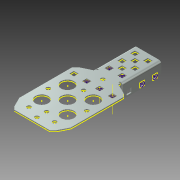
# Autodesk Inventor part: VEX_Bracket
Saved by Autodesk Inventor 2013 (Build 170138000, 138)
## iProperties
Created: 2011-03-28
Part Number: VEX_Bracket
Material: Aluminum-6061
Document SubType Name: Sheet Metal
Designer: Phillip
Density: 2.71 g/cm^3
Sheet Metal Rule: Default
Mass: 13.8705 g
Surface Area: 99.2536 cm^2
Volume: 5.11826 cm^3
Flat Pattern Width: 5.08 cm
Flat Pattern Length: 11.43 cm
Flat Pattern Area: 58.0644 cm^2
Sheet Metal Width: 2.000 in
Sheet Metal Length: 4.500 in
Sheet Metal Area: 9.000 in^2
Author: Phillip
Autodesk Inventor part; units mm, degrees
ref_plane "YZ Plane" through (0, 0, 0) normal (1, 0, 0) x (0, 1, 0)
ref_plane "XZ Plane" through (0, 0, 0) normal (0, 1, 0) x (-1, 0, 0)
ref_plane "XY Plane" through (0, 0, 0) normal (0, 0, 1) x (1, 0, 0)
sketch "Sketch1" plane through (0, 0, 0) normal (0, 0, 1) x (1, 0, 0)
  line L0 (-3.175, 3.175) -> (-7.9375, 12.7)
  line L1 (-3.175, 3.175) -> (0, 0)
  line L2 (0, 0) -> (34.925, 0)
  line L3 (38.1, 3.175) -> (34.925, 0)
  line L4 (38.1, 3.175) -> (42.8625, 12.7)
  line L5 (42.8625, 12.7) -> (42.8625, 65.0133)
  line L6 (39.6875, 68.1883) -> (42.8625, 65.0133)
  line L7 (39.6875, 68.1883) -> (29.5402, 73.025)
  line L8 (29.5402, 73.025) -> (29.5402, 114.3)
  line L9 (29.5402, 114.3) -> (5.3848, 114.3)
  line L10 (5.3848, 114.3) -> (5.3848, 73.025)
  line L11 (-4.7625, 68.1883) -> (5.3848, 73.025)
  line L12 (-4.7625, 68.1883) -> (-7.9375, 65.0133)
  line L13 (-7.9375, 12.7) -> (-7.9375, 65.0133)
  line L14 (19.7739, 99.2886) -> (19.7739, 103.9114)
  line L15 (15.1511, 99.2886) -> (19.7739, 99.2886)
  line L16 (15.1511, 103.9114) -> (15.1511, 99.2886)
  line L17 (19.7739, 103.9114) -> (15.1511, 103.9114)
  line L18 (13.4239, 105.6386) -> (13.4239, 110.2614)
  line L19 (8.8011, 105.6386) -> (13.4239, 105.6386)
  line L20 (8.8011, 110.2614) -> (8.8011, 105.6386)
  line L21 (13.4239, 110.2614) -> (8.8011, 110.2614)
  line L22 (26.1239, 105.6386) -> (26.1239, 110.2614)
  line L23 (21.5011, 105.6386) -> (26.1239, 105.6386)
  line L24 (21.5011, 110.2614) -> (21.5011, 105.6386)
  line L25 (26.1239, 110.2614) -> (21.5011, 110.2614)
  line L26 (26.1239, 58.0136) -> (26.1239, 62.6364)
  line L27 (21.5011, 58.0136) -> (26.1239, 58.0136)
  line L28 (21.5011, 62.6364) -> (21.5011, 58.0136)
  line L29 (26.1239, 62.6364) -> (21.5011, 62.6364)
  line L30 (38.8239, 58.0136) -> (38.8239, 62.6364)
  line L31 (34.2011, 58.0136) -> (38.8239, 58.0136)
  line L32 (34.2011, 62.6364) -> (34.2011, 58.0136)
  line L33 (38.8239, 62.6364) -> (34.2011, 62.6364)
  circle A0 centre (30.1625, 47.625) radius 6.35
  circle A1 centre (4.7625, 47.625) radius 6.35
  circle A2 centre (4.7625, 22.225) radius 6.35
  circle A3 centre (30.1625, 22.225) radius 6.35
  circle A4 centre (17.4625, 34.925) radius 6.35
  circle A5 centre (17.4625, 69.85) radius 2.0701
  circle A6 centre (17.4625, 50.8) radius 2.0701
  circle A7 centre (17.4625, 14.2875) radius 2.0701
  circle A8 centre (17.4625, 4.7625) radius 2.0701
  circle A9 centre (4.7625, 9.525) radius 2.0701
  circle A10 centre (30.1625, 9.525) radius 2.0701
  circle A11 centre (-1.5875, 34.925) radius 2.0701
  circle A12 centre (36.5125, 34.925) radius 2.0701
  line L34 (13.4239, 58.0136) -> (13.4239, 62.6364)
  line L35 (8.8011, 58.0136) -> (13.4239, 58.0136)
  line L36 (8.8011, 62.6364) -> (8.8011, 58.0136)
  line L37 (13.4239, 62.6364) -> (8.8011, 62.6364)
  line L38 (0.7239, 58.0136) -> (0.7239, 62.6364)
  line L39 (-3.8989, 58.0136) -> (0.7239, 58.0136)
  line L40 (-3.8989, 62.6364) -> (-3.8989, 58.0136)
  line L41 (0.7239, 62.6364) -> (-3.8989, 62.6364)
  line L42 (26.1239, 92.9386) -> (26.1239, 97.5614)
  line L43 (21.5011, 92.9386) -> (26.1239, 92.9386)
  line L44 (21.5011, 97.5614) -> (21.5011, 92.9386)
  line L45 (26.1239, 97.5614) -> (21.5011, 97.5614)
  line L46 (13.4239, 92.9386) -> (13.4239, 97.5614)
  line L47 (8.8011, 92.9386) -> (13.4239, 92.9386)
  line L48 (8.8011, 97.5614) -> (8.8011, 92.9386)
  line L49 (13.4239, 97.5614) -> (8.8011, 97.5614)
  line L50 (26.1239, 80.2386) -> (26.1239, 84.8614)
  line L51 (21.5011, 80.2386) -> (26.1239, 80.2386)
  line L52 (21.5011, 84.8614) -> (21.5011, 80.2386)
  line L53 (26.1239, 84.8614) -> (21.5011, 84.8614)
  line L54 (13.4239, 80.2386) -> (13.4239, 84.8614)
  line L55 (8.8011, 80.2386) -> (13.4239, 80.2386)
  line L56 (8.8011, 84.8614) -> (8.8011, 80.2386)
  line L57 (13.4239, 84.8614) -> (8.8011, 84.8614)
  line L58 (19.7739, 86.5886) -> (19.7739, 91.2114)
  line L59 (15.1511, 86.5886) -> (19.7739, 86.5886)
  line L60 (15.1511, 91.2114) -> (15.1511, 86.5886)
  line L61 (19.7739, 91.2114) -> (15.1511, 91.2114)
  circle A13 centre (11.1125, 107.95) radius 2.3114
  circle A14 centre (11.1125, 95.25) radius 2.3114
  circle A15 centre (11.1125, 82.55) radius 2.3114
  circle A16 centre (23.8125, 107.95) radius 2.3114
  circle A17 centre (23.8125, 95.25) radius 2.3114
  circle A18 centre (23.8125, 82.55) radius 2.3114
  circle A19 centre (-1.5875, 60.325) radius 2.3114
  circle A20 centre (11.1125, 60.325) radius 2.3114
  circle A21 centre (23.8125, 60.325) radius 2.3114
  circle A22 centre (36.5125, 60.325) radius 2.3114
  dimension "d8" = 12.7
  dimension "d9" = 12.7
  dimension "d10" = 12.7
  dimension "d12" = 6.35
  dimension "d13" = 24.1554
  dimension "d14" = 41.275
  dimension "d15" = 114.3
  dimension "d16" = 50.8
  dimension "d17" = 4.1402
  dimension "d18" = 4.6228
  dimension "d19" = 4.6228
  measures "d8" distance of A13.centre A14.centre
  measures "d9" distance of A13.centre A16.centre
  measures "d10" distance of A19.centre A20.centre
  measures "d12" distance from line of A13.centre L9
  measures "d13" distance of L8.end L10.start
  measures "d14" distance of L8.start L8.end
  measures "d15" vertical distance of L3.end L8.end
  measures "d16" distance between parallel lines of L5 L13
  measures "d17" diameter of A11
  measures "d18" distance of L57.end L56.end
  measures "d19" distance of L57.start L57.end
extrude "Plate1" add sketch "Sketch1" along normal blind 1.1684
sketch "Sketch2" plane through (29.5402, 73.025, 0) normal (1, 0, 0) x (0, 0, -1)
  line L0 (0, 41.275) -> (12.7, 41.275)
  line L1 (12.7, 41.275) -> (12.7, 3.175)
  line L2 (12.7, 3.175) -> (0, 3.175)
  line L3 (0, 3.175) -> (0, 41.275)
  point P0 (0, -73.025)
  dimension "d21" = 12.7
  dimension "d22" = 38.1
  measures "d21" distance of L1.end L2.end
  measures "d22" distance of L0.end L1.end
sheet face with bend "Face2" sketch "Sketch2" thickness 1.1684 toward (1, 0, 0) bend radius 1.1684 relief straight relief width 1.1684 relief depth 0.5842
bend "Bend1"
sketch "Sketch3" plane through (5.3848, 73.025, 0) normal (-1, 0, 0) x (0, 0, 1)
  line L0 (0, 41.275) -> (-12.7, 41.275)
  line L1 (-12.7, 41.275) -> (-12.7, 3.175)
  line L2 (-12.7, 3.175) -> (0, 3.175)
  line L3 (0, 3.175) -> (0, 41.275)
  point P0 (0, -73.025)
  dimension "d28" = 12.7
  dimension "d29" = 38.1
  measures "d28" distance of L2.end L1.end
  measures "d29" distance of L1.end L0.end
sheet face with bend "Face3" sketch "Sketch3" thickness 1.1684 toward (-1, 0, 0) bend radius 1.1684 relief straight relief width 1.1684 relief depth 0.5842
bend "Bend2"
sketch "Sketch4" plane through (30.7086, 73.025, 0) normal (1, 0, 0) x (0, 0, -1)
  line L0 (1.1684, 41.275) -> (1.1684, 3.175)
  line L1 (11.2522, 37.2364) -> (6.6294, 37.2364)
  line L2 (11.2522, 32.6136) -> (11.2522, 37.2364)
  line L3 (6.6294, 32.6136) -> (11.2522, 32.6136)
  line L4 (6.6294, 37.2364) -> (6.6294, 32.6136)
  line L5 (11.2522, 24.5364) -> (6.6294, 24.5364)
  line L6 (11.2522, 19.9136) -> (11.2522, 24.5364)
  line L7 (6.6294, 19.9136) -> (11.2522, 19.9136)
  line L8 (6.6294, 24.5364) -> (6.6294, 19.9136)
  line L9 (11.2522, 11.8364) -> (6.6294, 11.8364)
  line L10 (11.2522, 7.2136) -> (11.2522, 11.8364)
  line L11 (6.6294, 7.2136) -> (11.2522, 7.2136)
  line L12 (6.6294, 11.8364) -> (6.6294, 7.2136)
  point P0 (0, -73.025)
  constraints: 26 end point
extrude "Cut1" cut sketch "Sketch4" against normal blind 1.1684
chamfer "Corner Chamfer1" distance 3.175 angle 45 4 edges at (30.1244, 114.3, -12.7) (30.1244, 76.2, -12.7) (4.8006, 76.2, -12.7) (4.8006, 114.3, -12.7)
sketch "Sketch5" plane through (4.2164, 73.025, 0) normal (-1, 0, 0) x (0, 0, 1)
  line L0 (-1.1684, 3.175) -> (-1.1684, 41.275)
  line L1 (-11.2522, 7.2136) -> (-6.6294, 7.2136)
  line L2 (-11.2522, 11.8364) -> (-11.2522, 7.2136)
  line L3 (-6.6294, 11.8364) -> (-11.2522, 11.8364)
  line L4 (-6.6294, 7.2136) -> (-6.6294, 11.8364)
  line L5 (-11.2522, 19.9136) -> (-6.6294, 19.9136)
  line L6 (-11.2522, 24.5364) -> (-11.2522, 19.9136)
  line L7 (-6.6294, 24.5364) -> (-11.2522, 24.5364)
  line L8 (-6.6294, 19.9136) -> (-6.6294, 24.5364)
  line L9 (-11.2522, 32.6136) -> (-6.6294, 32.6136)
  line L10 (-11.2522, 37.2364) -> (-11.2522, 32.6136)
  line L11 (-6.6294, 37.2364) -> (-11.2522, 37.2364)
  line L12 (-6.6294, 32.6136) -> (-6.6294, 37.2364)
  point P0 (0, -73.025)
  constraints: 26 end point
extrude "Cut2" cut sketch "Sketch5" against normal blind 1.1684
sketch "Sketch7" plane through (0, 0, 0) normal (0, 0, -1) x (-1, 0, 0)
  circle A0 centre (-4.7625, 22.225) radius 6.35 projected
  circle A1 centre (-17.4625, 34.925) radius 6.35 projected
  circle A2 centre (-4.7625, 47.625) radius 6.35 projected
  circle A3 centre (-30.1625, 22.225) radius 6.35 projected
  circle A4 centre (-30.1625, 47.625) radius 6.35 projected
  line L0 (-21.5011, 110.2614) -> (-21.5011, 105.6386) projected
  line L1 (-21.5011, 105.6386) -> (-26.1239, 105.6386) projected
  line L2 (-26.1239, 105.6386) -> (-26.1239, 110.2614) projected
  line L3 (-26.1239, 110.2614) -> (-21.5011, 110.2614) projected
  line L4 (-15.1511, 86.5886) -> (-19.7739, 86.5886) projected
  line L5 (-19.7739, 86.5886) -> (-19.7739, 91.2114) projected
  line L6 (-19.7739, 91.2114) -> (-15.1511, 91.2114) projected
  line L7 (-15.1511, 91.2114) -> (-15.1511, 86.5886) projected
  line L8 (-8.8011, 105.6386) -> (-13.4239, 105.6386) projected
  line L9 (-13.4239, 105.6386) -> (-13.4239, 110.2614) projected
  line L10 (-13.4239, 110.2614) -> (-8.8011, 110.2614) projected
  line L11 (-8.8011, 110.2614) -> (-8.8011, 105.6386) projected
  line L12 (-15.1511, 99.2886) -> (-19.7739, 99.2886) projected
  line L13 (-19.7739, 99.2886) -> (-19.7739, 103.9114) projected
  line L14 (-19.7739, 103.9114) -> (-15.1511, 103.9114) projected
  line L15 (-15.1511, 103.9114) -> (-15.1511, 99.2886) projected
  line L16 (-21.5011, 58.0136) -> (-26.1239, 58.0136) projected
  line L17 (-26.1239, 58.0136) -> (-26.1239, 62.6364) projected
  line L18 (-26.1239, 62.6364) -> (-21.5011, 62.6364) projected
  line L19 (-21.5011, 62.6364) -> (-21.5011, 58.0136) projected
  line L20 (-21.5011, 80.2386) -> (-26.1239, 80.2386) projected
  line L21 (-26.1239, 80.2386) -> (-26.1239, 84.8614) projected
  line L22 (-26.1239, 84.8614) -> (-21.5011, 84.8614) projected
  line L23 (-21.5011, 84.8614) -> (-21.5011, 80.2386) projected
  line L24 (-26.1239, 97.5614) -> (-21.5011, 97.5614) projected
  line L25 (-21.5011, 97.5614) -> (-21.5011, 92.9386) projected
  line L26 (-21.5011, 92.9386) -> (-26.1239, 92.9386) projected
  line L27 (-26.1239, 92.9386) -> (-26.1239, 97.5614) projected
  line L28 (-8.8011, 58.0136) -> (-13.4239, 58.0136) projected
  line L29 (-13.4239, 58.0136) -> (-13.4239, 62.6364) projected
  line L30 (-13.4239, 62.6364) -> (-8.8011, 62.6364) projected
  line L31 (-8.8011, 62.6364) -> (-8.8011, 58.0136) projected
  line L32 (-8.8011, 84.8614) -> (-8.8011, 80.2386) projected
  line L33 (-8.8011, 80.2386) -> (-13.4239, 80.2386) projected
  line L34 (-13.4239, 80.2386) -> (-13.4239, 84.8614) projected
  line L35 (-13.4239, 84.8614) -> (-8.8011, 84.8614) projected
  line L36 (-8.8011, 97.5614) -> (-8.8011, 92.9386) projected
  line L37 (-8.8011, 92.9386) -> (-13.4239, 92.9386) projected
  line L38 (-13.4239, 92.9386) -> (-13.4239, 97.5614) projected
  line L39 (-13.4239, 97.5614) -> (-8.8011, 97.5614) projected
  line L40 (-34.2011, 58.0136) -> (-38.8239, 58.0136) projected
  line L41 (-38.8239, 58.0136) -> (-38.8239, 62.6364) projected
  line L42 (-38.8239, 62.6364) -> (-34.2011, 62.6364) projected
  line L43 (-34.2011, 62.6364) -> (-34.2011, 58.0136) projected
  line L44 (3.8989, 58.0136) -> (-0.7239, 58.0136) projected
  line L45 (-0.7239, 58.0136) -> (-0.7239, 62.6364) projected
  line L46 (-0.7239, 62.6364) -> (3.8989, 62.6364) projected
  line L47 (3.8989, 62.6364) -> (3.8989, 58.0136) projected
  circle A5 centre (1.5875, 34.925) radius 2.0701 projected
  circle A6 centre (-36.5125, 34.925) radius 2.0701 projected
  circle A7 centre (-17.4625, 50.8) radius 2.0701 projected
  circle A8 centre (-17.4625, 69.85) radius 2.0701 projected
  circle A9 centre (-17.4625, 14.2875) radius 2.0701 projected
  circle A10 centre (-30.1625, 9.525) radius 2.0701 projected
  circle A11 centre (-17.4625, 4.7625) radius 2.0701 projected
  circle A12 centre (-4.7625, 9.525) radius 2.0701 projected
  line L48 (-5.3848, 75.0316) -> (-7.1374, 75.0316) projected
  line L49 (-7.1374, 75.0316) -> (-7.1374, 76.2) projected
  line L50 (-7.1374, 76.2) -> (-6.5532, 76.2) projected
  line L51 (-6.5532, 76.2) -> (-6.5532, 114.3) projected
  line L52 (-28.3718, 114.3) -> (-6.5532, 114.3) projected
  line L53 (-28.3718, 114.3) -> (-28.3718, 76.2) projected
  line L54 (-28.3718, 76.2) -> (-27.7876, 76.2) projected
  line L55 (-27.7876, 76.2) -> (-27.7876, 75.0316) projected
  line L56 (-27.7876, 75.0316) -> (-29.5402, 75.0316) projected
  line L57 (-29.5402, 73.025) -> (-29.5402, 75.0316) projected
  line L58 (-39.6875, 68.1883) -> (-29.5402, 73.025) projected
  line L59 (-42.8625, 65.0133) -> (-39.6875, 68.1883) projected
  line L60 (-42.8625, 12.7) -> (-42.8625, 65.0133) projected
  line L61 (-38.1, 3.175) -> (-42.8625, 12.7) projected
  line L62 (-34.925, 0) -> (-38.1, 3.175) projected
  line L63 (0, 0) -> (-34.925, 0) projected
  line L64 (3.175, 3.175) -> (0, 0) projected
  line L65 (7.9375, 12.7) -> (3.175, 3.175) projected
  line L66 (7.9375, 65.0133) -> (7.9375, 12.7) projected
  line L67 (4.7625, 68.1883) -> (7.9375, 65.0133) projected
  line L68 (-5.3848, 73.025) -> (4.7625, 68.1883) projected
  line L69 (-5.3848, 75.0316) -> (-5.3848, 73.025) projected
  circle A13 centre (-23.8125, 82.55) radius 2.3114
  circle A14 centre (-11.1125, 82.55) radius 2.3114
  constraints: 8 tangent, 2 centre point
sketch "Sketch8" plane through (0, 0, 0) normal (0, 0, -1) x (-1, 0, 0)
  line L0 (-21.5011, 58.0136) -> (-26.1239, 58.0136) projected
  line L1 (-26.1239, 58.0136) -> (-26.1239, 62.6364) projected
  line L2 (-26.1239, 62.6364) -> (-21.5011, 62.6364) projected
  line L3 (-21.5011, 62.6364) -> (-21.5011, 58.0136) projected
  line L4 (-34.2011, 58.0136) -> (-38.8239, 58.0136) projected
  line L5 (-38.8239, 58.0136) -> (-38.8239, 62.6364) projected
  line L6 (-38.8239, 62.6364) -> (-34.2011, 62.6364) projected
  line L7 (-34.2011, 62.6364) -> (-34.2011, 58.0136) projected
  circle A0 centre (-36.5125, 60.325) radius 2.3114
  circle A1 centre (-23.8125, 60.325) radius 2.3114
  line L8 (-8.8011, 58.0136) -> (-13.4239, 58.0136) projected
  line L9 (-13.4239, 58.0136) -> (-13.4239, 62.6364) projected
  line L10 (-13.4239, 62.6364) -> (-8.8011, 62.6364) projected
  line L11 (-8.8011, 62.6364) -> (-8.8011, 58.0136) projected
  circle A2 centre (-11.1125, 60.325) radius 2.3114
  constraints: 12 tangent, 3 centre point
surface extrude "ExtrusionSrf1" sketch "Sketch8" against normal up to surface (1.1684 mm away) shown no curves A0
surface extrude "ExtrusionSrf2" sketch "Sketch8" against normal up to surface (1.1684 mm away) shown no curves A1
surface extrude "ExtrusionSrf3" sketch "Sketch8" against normal up to surface (1.1684 mm away) shown no curves A2
sketch "Sketch9" plane through (30.7086, 73.025, 0) normal (1, 0, 0) x (0, 0, -1)
  line L0 (11.2522, 37.2364) -> (11.2522, 32.6136) projected
  line L1 (11.2522, 32.6136) -> (6.6294, 32.6136) projected
  line L2 (6.6294, 32.6136) -> (6.6294, 37.2364) projected
  line L3 (6.6294, 37.2364) -> (11.2522, 37.2364) projected
  line L4 (6.6294, 24.5364) -> (11.2522, 24.5364) projected
  line L5 (11.2522, 24.5364) -> (11.2522, 19.9136) projected
  line L6 (11.2522, 19.9136) -> (6.6294, 19.9136) projected
  line L7 (6.6294, 19.9136) -> (6.6294, 24.5364) projected
  circle A0 centre (8.9408, 22.225) radius 2.3114
  circle A1 centre (8.9408, 34.925) radius 2.3114
  point P0 (0, -73.025)
  constraints: 8 tangent, 2 centre point
surface extrude "ExtrusionSrf4" sketch "Sketch9" against normal up to surface (1.1684 mm away) shown no curves A0
surface extrude "ExtrusionSrf5" sketch "Sketch9" against normal up to surface (1.1684 mm away) shown no curves A1
equation "\"d35\" = Thickness"
equation "\"d40\" = Thickness"
equation "\"d23\" = BendRadius"
equation "\"d24\" = BendReliefWidth"
equation "\"d26\" = MinimumRemnant"
equation "\"d25\" = BendReliefDepth"
equation "\"d27\" = BendRadius"
equation "\"d30\" = BendRadius"
equation "\"d31\" = BendReliefWidth"
equation "\"d33\" = MinimumRemnant"
equation "\"d32\" = BendReliefDepth"
equation "\"d34\" = BendRadius"
equation "\"BendRadius\" = Thickness"
equation "\"BendReliefWidth\" = Thickness"
equation "\"BendReliefDepth\" = 0.5 * Thickness"
equation "\"CornerReliefSize\" = 4 * Thickness"
equation "\"MinimumRemnant\" = 2 * Thickness"
equation "\"TransitionRadius\" = BendRadius"
equation "\"JacobiRadiusSize\" = BendRadius"
equation "\"GapSize\" = Thickness"
equation "\"d20\" = BendRadius"
equation "\"Thickness\" = 1.1684"
body "Solid1"
body "Srf1"
body "Srf2"
body "Srf3"
body "Srf4"
body "Srf5"
